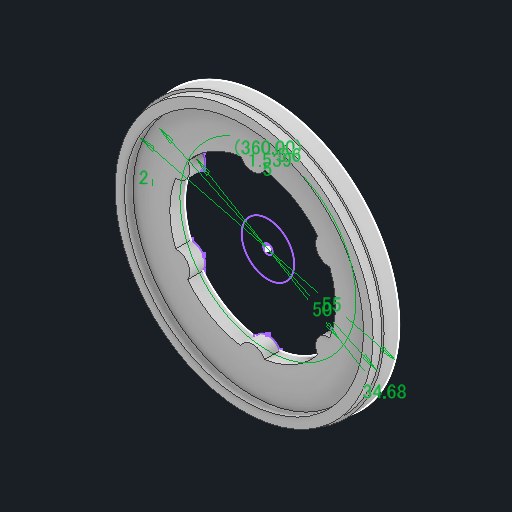
# Autodesk Inventor part: baicPart
Saved by Autodesk Inventor 2025.2 (Build 292293000, 293)
## iProperties
Company: FC-TORQUE
Created: 2025-03-14
Part Number: baicPart
Material: 一般
Document SubType Name: Modeling
Designer: Keito Tamura
Density: 1 g/cm^3
Appearance: 既定
Author: Keito Tamura
Autodesk Inventor part; units mm, degrees
ref_plane "YZ Plane" through (0, 0, 0) normal (1, 0, 0) x (0, 1, 0)
ref_plane "XZ Plane" through (0, 0, 0) normal (0, 1, 0) x (-1, 0, 0)
ref_plane "XY Plane" through (0, 0, 0) normal (0, 0, 1) x (1, 0, 0)
sketch "スケッチ1" plane through (0, 0, 0) normal (0, 0, 1) x (1, 0, 0)
  circle A0 centre (0, 0) radius 17.34
  circle A1 centre (0, 0) radius 5.5
  circle A2 centre (0, 0) radius 18.4198
  circle A3 centre (0, 18.4198) radius 2.8
  line L0 (-2.5, 17.1588) -> (2.5, 17.1588)
  line L1 (0, 15.6198) -> (0, 17.1588)
  circle A4 centre (-15.952, 9.2099) radius 2.8
  circle A5 centre (-15.952, -9.2099) radius 2.8
  circle A6 centre (0, -18.4198) radius 2.8
  circle A7 centre (15.952, -9.2099) radius 2.8
  circle A8 centre (15.952, 9.2099) radius 2.8
  circle A9 centre (0, 0) radius 0.9862
  circle A10 centre (0, 0) radius 25
  circle A11 centre (0, 0) radius 27
  circle A12 centre (0, 0) radius 27.5
  point P0 (-0.3987, 0.1519)
  point P1 (-0.3987, 0.1519)
  point P2 (-0.3987, 0.1519)
  point P3 (-0.3987, 0.1519)
  point P4 (-0.3987, 0.1519)
  point P5 (-0.3987, 0.1519)
  point P6 (-0.3987, 0.1519)
  point P7 (-0.3987, 0.1519)
  point P8 (-0.3987, 0.1519)
  point P9 (-0.3987, 0.1519)
  point P10 (-0.3987, 0.1519)
  point P11 (-0.3987, 0.1519)
  point P12 (-0.3987, 0.1519)
  point P13 (-0.3987, 0.1519)
  point P14 (-0.3987, 0.1519)
  point P15 (-0.3987, 0.1519)
  point P16 (-0.3987, 0.1519)
  point P17 (-0.3987, 0.1519)
  point P18 (-0.3987, 0.1519)
  point P19 (-0.3987, 0.1519)
  point P20 (-0.3987, 0.1519)
  point P21 (-0.3987, 0.1519)
  point P22 (-0.3987, 0.1519)
  point P23 (-0.3987, 0.1519)
  point P24 (-0.3987, 0.1519)
  point P25 (-0.3987, 0.1519)
  point P26 (-0.3987, 0.1519)
  point P27 (-0.3987, 0.1519)
  point P28 (-0.3987, 0.1519)
  point P29 (-0.3987, 0.1519)
  point P30 (-0.3987, 0.1519)
  point P31 (-0.3987, 0.1519)
  point P32 (-0.3987, 0.1519)
  point P33 (-0.3987, 0.1519)
  point P34 (-0.3987, 0.1519)
  point P35 (-0.3987, 0.1519)
  point P36 (-0.3987, 0.1519)
  point P37 (-0.3987, 0.1519)
  point P38 (-0.3987, 0.1519)
  point P39 (-0.3987, 0.1519)
  point P40 (-0.3987, 0.1519)
  point P41 (-0.3987, 0.1519)
  point P42 (-0.3987, 0.1519)
  point P43 (-0.3987, 0.1519)
  point P44 (-0.3987, 0.1519)
  point P45 (-0.3987, 0.1519)
  point P46 (-0.3987, 0.1519)
  point P47 (-0.3987, 0.1519)
  point P48 (-0.3987, 0.1519)
  point P49 (-0.3987, 0.1519)
  point P50 (-0.3987, 0.1519)
  point P51 (-0.3987, 0.1519)
  point P52 (-0.3987, 0.1519)
  point P53 (-0.3987, 0.1519)
  point P54 (-0.3987, 0.1519)
  point P55 (-0.3987, 0.1519)
  point P56 (-0.3987, 0.1519)
  point P57 (-0.3987, 0.1519)
  point P58 (-0.3987, 0.1519)
  point P59 (-0.3987, 0.1519)
  point P60 (-0.3987, 0.1519)
  point P61 (-0.3987, 0.1519)
  point P62 (-0.3987, 0.1519)
  point P63 (-0.3987, 0.1519)
  point P64 (-0.3987, 0.1519)
  point P65 (-0.3987, 0.1519)
  point P66 (-0.3987, 0.1519)
  point P67 (-0.3987, 0.1519)
  point P68 (-0.3987, 0.1519)
  point P69 (-0.3987, 0.1519)
  point P70 (-0.3987, 0.1519)
  point P71 (-0.3987, 0.1519)
  point P72 (-0.3987, 0.1519)
  point P73 (-0.3987, 0.1519)
  point P74 (-0.3987, 0.1519)
  point P75 (-16.11, 6.4144)
  point P76 (-13.61, 10.7445)
  point P77 (-13.5271, 7.8099)
  point P78 (-13.61, -10.7445)
  point P79 (-16.11, -6.4144)
  point P80 (-13.5271, -7.8099)
  point P81 (2.5, -17.1588)
  point P82 (-2.5, -17.1588)
  point P83 (0, -15.6198)
  point P84 (16.11, -6.4144)
  point P85 (13.61, -10.7445)
  point P86 (13.5271, -7.8099)
  point P87 (13.61, 10.7445)
  point P88 (16.11, 6.4144)
  point P89 (13.5271, 7.8099)
  point P90 (16.11, 6.4144)
  point P91 (16.11, -6.4144)
  point P92 (13.61, -10.7445)
  point P93 (2.5, -17.1588)
  point P94 (-2.5, -17.1588)
  point P95 (-13.61, -10.7445)
  point P96 (-16.11, -6.4144)
  point P97 (-16.11, 6.4144)
  point P98 (-13.61, 10.7445)
  point P99 (13.61, 10.7445)
  dimension "d2" = 34.68
  dimension "d3" = 5.6
  dimension "d4" = 5
  dimension "d5" = 1.5391
  dimension "d6" = 360
  dimension "d7" = 50
  dimension "d8" = 2
  dimension "d9" = 55
  constraints: 20 point on circle, 12 centre point, 10 coincident, 4 end point, 2 concentric, 1 midpoint, 34 other
  measures "d2" diameter of A0
  measures "d3" diameter of A3
  measures "d4" distance of L0.start L0.end
  measures "d5" distance of L1.start L1.end
  measures "d7" diameter of A10
  measures "d8" radial gap between concentric circles of A10 A11
  measures "d9" diameter of A12
extrude "押し出し1" add sketch "スケッチ1" along normal blind 3.2 contours L0 A0 | A3 A2 A8 A0 | A0 A3 A2 | A3 L1 L0 | L0 L1 A3 | A0 A4 A2 A3 | A8 A2 A0 | A0 A8 | A2 A3 | A4 A0 | A0 A4 A2 | A8 A2 A7 A0 | A8 A2 | A0 A5 A2 A4 | A2 A4 | A5 A0 | A0 A5 A2 | A7 A2 A0 | A0 A7 | A0 A6 A2 A5 | A2 A5 | A7 A2 A6 A0 | A7 A2 | A6 A0 | A0 A6 A2 | A2 A6 | A10 | A12
extrude "押し出し2" add sketch "スケッチ1" along normal blind 5 contours A11
